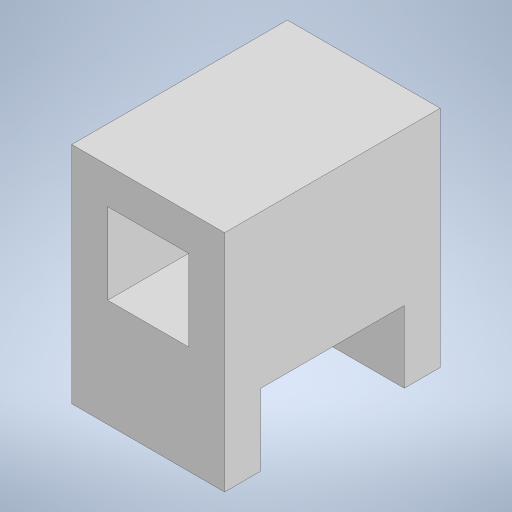
# Autodesk Inventor part: zigu3
Saved by Autodesk Inventor 2024.3 (Build 283343010, 343A)
## iProperties
Created: 2025-10-22
Part Number: zigu3
Material: 一般
Document SubType Name: Modeling
Designer: kshau
Density: 1 g/cm^3
Appearance: 既定
Author: kshau
Autodesk Inventor part; units mm, degrees
ref_plane "YZ Plane" through (0, 0, 0) normal (1, 0, 0) x (0, 1, 0)
ref_plane "XZ Plane" through (0, 0, 0) normal (0, 1, 0) x (-1, 0, 0)
ref_plane "XY Plane" through (0, 0, 0) normal (0, 0, 1) x (1, 0, 0)
sketch "スケッチ1" plane through (0, 0, 0) normal (0, 0, 1) x (1, 0, 0)
  line L0 (0, 0) -> (42.6, 0)
  line L1 (42.6, 0) -> (42.6, 42.6)
  line L2 (42.6, 42.6) -> (0, 42.6)
  line L3 (0, 42.6) -> (0, 0)
  line L4 (10, 32.6) -> (32.6, 32.6)
  line L5 (32.6, 32.6) -> (32.6, 10)
  line L6 (32.6, 10) -> (10, 10)
  line L7 (10, 10) -> (10, 32.6)
  dimension "d0" = 42.6
  dimension "d1" = 42.6
  dimension "d2" = 10
  dimension "d3" = 10
  dimension "d4" = 10
  dimension "d5" = 10
  constraints: 16 end point, 4 parallel, 2 horizontal, 2 perpendicular
  measures "d0" distance of L0.end L1.end
  measures "d1" distance of L1.end L2.end
  measures "d2" distance between parallel lines of L3 L7
  measures "d3" distance between parallel lines of L1 L5
  measures "d4" distance between parallel lines of L0 L6
  measures "d5" distance between parallel lines of L2 L4
extrude "押し出し1" add sketch "スケッチ1" along normal blind 20.05
sketch "スケッチ2" plane through (0, 0, 20.05) normal (0, 0, 1) x (1, 0, 0)
  line L0 (10, 10) -> (10, 32.6) projected
  line L1 (32.6, 32.6) -> (32.6, 10) projected
  line L2 (10, 10) -> (32.6, 10)
  line L3 (32.6, 10) -> (32.6, 32.6)
  line L4 (32.6, 32.6) -> (10, 32.6)
  line L5 (10, 32.6) -> (10, 10)
  line L6 (42.6, 42.6) -> (0, 42.6) projected
  line L7 (0, 42.6) -> (42.6, 42.6)
  line L8 (42.6, 42.6) -> (42.6, -20)
  line L9 (42.6, -20) -> (0, -20)
  line L10 (0, -20) -> (0, 42.6)
  line L11 (0, 0) -> (42.6, 0) projected
  dimension "d8" = 20
  constraints: 16 end point, 4 parallel, 2 horizontal, 2 perpendicular, 1 point on line
  measures "d8" distance between parallel lines of L11 L9
extrude "押し出し2" add sketch "スケッチ2" along normal blind 10
mirror "ミラー1" about plane through (21.3, 21.3, 0) normal (0, 0, -1) of "押し出し1", "押し出し2"
